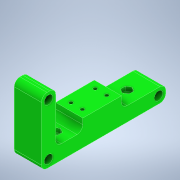
# Autodesk Inventor part: wheel_mount
Saved by Autodesk Inventor 2021 (Build 250183000, 183)
## iProperties
Created: 2022-05-16
Part Number: wheel_mount
Material: Generic
Document SubType Name: Modeling
Designer: ermoz
Density: 1 g/cm^3
Appearance: Default
Author: ermoz
Autodesk Inventor part; units mm, degrees
ref_plane "YZ Plane" through (0, 0, 0) normal (1, 0, 0) x (0, 1, 0)
ref_plane "XZ Plane" through (0, 0, 0) normal (0, 1, 0) x (-1, 0, 0)
ref_plane "XY Plane" through (0, 0, 0) normal (0, 0, 1) x (1, 0, 0)
sketch "Sketch1" plane through (0, 0, 0) normal (1, 0, 0) x (0, 1, 0)
  circle A0 centre (0, 0) radius 3
  circle A1 centre (0, 77) radius 3
  circle A2 centre (36, 77) radius 3
  line L0 (-5, 78) -> (-5, -1)
  line L1 (-1, 82) -> (37, 82)
  line L2 (41, 78) -> (41, 76)
  line L3 (37, 72) -> (9, 72)
  line L4 (5, 68) -> (5, -1)
  line L5 (36, 77) -> (41, 77)
  line L6 (0, 0) -> (0, -5)
  line L7 (0, -5) -> (1, -5)
  line L8 (-1, -5) -> (0, -5)
  arc A3 (-1, 82) -> (-5, 78) centre (-1, 78) ccw
  arc A4 (-5, -1) -> (-1, -5) centre (-1, -1) ccw
  arc A5 (1, -5) -> (5, -1) centre (1, -1) ccw
  arc A6 (9, 72) -> (5, 68) centre (9, 68) ccw
  arc A7 (37, 72) -> (41, 76) centre (37, 76) ccw
  arc A8 (41, 78) -> (37, 82) centre (37, 78) ccw
  dimension "d0" = 6
  dimension "d1" = 77
  dimension "d3" = 10
  dimension "d4" = 5
  dimension "d5" = 4
  dimension "d6" = 10
  dimension "d9" = 46
  constraints: 18 end point, 12 point on circle, 12 tangent, 9 centre point, 7 equal radius, 3 horizontal, 3 perpendicular, 2 equal length, 2 horizontal alignment, 2 vertical alignment, 1 coincident, 1 collinear, 1 midpoint, 1 vertical
  measures "d0" diameter of A0
  measures "d1" distance of A1.centre point (0, 0)
  measures "d3" distance between parallel lines of L1 L3
  measures "d4" distance of L5.start L5.end
  measures "d5" radius of A3
  measures "d6" distance between parallel lines of L0 L4
  measures "d9" distance between parallel lines of L2 L0
extrude "Extrusion1" add sketch "Sketch1" along normal blind 19
sketch "Sketch3" plane through (0, 5, -1) normal (0, 1, 0) x (1, 0, 0)
  line L0 (19, 0) -> (19, -69) projected
  line L1 (19, -27) -> (0, -27)
  line L2 (0, -27) -> (0, -54)
  line L3 (0, -54) -> (19, -54)
  line L4 (19, -54) -> (19, -27)
  line L5 (0, 4) -> (19, 4) projected
  line L6 (0, -83) -> (19, -83) projected
  line L7 (0, 0) -> (0, -69) projected
  point P0 (0, -1)
  point P1 (19, -54)
  dimension "d15" = 31
  dimension "d16" = 29
  constraints: 8 end point, 2 parallel, 1 collinear, 1 horizontal, 1 perpendicular, 1 point on line
  measures "d15" distance between parallel lines of L5 L1
  measures "d16" distance between parallel lines of L6 L3
extrude "Extrusion3" add sketch "Sketch3" along normal blind 8
fillet "Fillet1" radius 4 2 edges at (9.5, 5, 53) (9.5, 5, 26)
sketch "Sketch4" plane through (0, 5, -1) normal (0, 1, 0) x (1, 0, 0)
  line L0 (12.5, -15.2321) -> (9.5, -16.9641)
  line L1 (9.5, -16.9641) -> (6.5, -15.2321)
  line L2 (6.5, -15.2321) -> (6.5, -11.7679)
  line L3 (6.5, -11.7679) -> (9.5, -10.0359)
  line L4 (9.5, -10.0359) -> (12.5, -11.7679)
  line L5 (12.5, -11.7679) -> (12.5, -15.2321)
  line L6 (12.5, -65.2321) -> (9.5, -66.9641)
  line L7 (9.5, -66.9641) -> (6.5, -65.2321)
  line L8 (6.5, -65.2321) -> (6.5, -61.7679)
  line L9 (6.5, -61.7679) -> (9.5, -60.0359)
  line L10 (9.5, -60.0359) -> (12.5, -61.7679)
  line L11 (12.5, -61.7679) -> (12.5, -65.2321)
  line L12 (19, -58) -> (19, -69) projected
  line L13 (19, 0) -> (19, -23) projected
  line L14 (19, -23) -> (0, -23) projected
  line L15 (19, -27) -> (0, -27) projected
  line L16 (0, -54) -> (19, -54) projected
  circle A0 centre (9.5, -13.5) radius 1.5
  circle A1 centre (9.5, -63.5) radius 1.5
  point P0 (0, -1)
  point P1 (9.5, -23)
  dimension "d20" = 6
  dimension "d23" = 9.5
  dimension "d26" = 3
  dimension "d29" = 50
  constraints: 24 end point, 2 centre point, 2 coincident, 2 parallel, 2 vertical alignment, 1 equal radius, 1 midpoint, 1 point on line, 26 other
  measures "d20" distance between parallel lines of L0 L3
  measures "d23" distance from line of L16 point (9.5, -63.5)
  measures "d26" diameter of A0
  measures "d29" distance of point (9.5, -63.5) point (9.5, -13.5)
extrude "Extrusion4" cut sketch "Sketch4" against normal blind 3 contours L0 L1 L2 L3 L4 L5 | L6 L7 L8 L9 L10 L11 | A0 | A1
extrude "Extrusion5" cut sketch "Sketch4" against normal through all contours A0 | A1
sketch "Sketch5" plane through (0, 13, -1) normal (0, 1, 0) x (1, 0, 0)
  circle A0 centre (5.5, -31.8771) radius 1.25
  circle A1 centre (5.5, -48.8771) radius 1.25
  circle A2 centre (13.5, -31.8771) radius 1.25
  circle A3 centre (13.5, -48.8771) radius 1.25
  line L0 (19, -54) -> (19, -27) projected
  line L1 (0, -27) -> (0, -54) projected
  point P0 (0, -1)
  dimension "d30" = 2.5
  dimension "d31" = 17
  dimension "d32" = 5.5
  dimension "d33" = 5.5
  constraints: 4 centre point, 3 equal radius, 2 horizontal alignment, 2 vertical alignment
  measures "d30" diameter of A2
  measures "d31" distance of A3.centre A2.centre
  measures "d32" distance from line of L0 A2.centre
  measures "d33" distance from line of L1 A0.centre
extrude "Extrusion6" cut sketch "Sketch5" against normal through all
equation "\"d33\" = d32"
body "Solid1"
